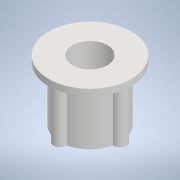
# Autodesk Inventor part: Tapa
Saved by Autodesk Inventor 2022 (Build 260153000, 153)
## iProperties
Created: 2022-08-23
Part Number: Tapa
Material: Generic
Document SubType Name: Modeling
Designer: David
Density: 1 g/cm^3
Appearance: Default
Author: David
Autodesk Inventor part; units mm, degrees
ref_plane "YZ Plane" through (0, 0, 0) normal (1, 0, 0) x (0, 1, 0)
ref_plane "XZ Plane" through (0, 0, 0) normal (0, 1, 0) x (-1, 0, 0)
ref_plane "XY Plane" through (0, 0, 0) normal (0, 0, 1) x (1, 0, 0)
sketch "Sketch8" plane through (0, 0, 0) normal (0, 1, 0) x (-1, 0, 0)
  circle A0 centre (0, 0) radius 13
  dimension "d25" = 26
  constraints: 1 centre point, 1 coincident
  measures "d25" diameter of A0
extrude "Extrusion8" add sketch "Sketch8" along normal blind 2
sketch "Sketch9" plane through (0, 0, 0) normal (0, -1, 0) x (1, 0, 0)
  circle A0 centre (0, 0) radius 9.5
  dimension "d28" = 19
  constraints: 1 centre point, 1 coincident
  measures "d28" diameter of A0
extrude "Extrusion9" add sketch "Sketch9" along normal blind 3
sketch "Sketch10" plane through (0, -3, 0) normal (0, -1, 0) x (1, 0, 0)
  circle A0 centre (0, 0) radius 9.5 projected
  circle A1 centre (-9.5, 0) radius 2
  line L0 (-18.2, 0) -> (18.2, 0) projected
  point P0 (-9.2895, -1.9889)
  point P1 (-9.2895, 1.9889)
  dimension "d31" = 4
  constraints: 1 centre point, 1 point on line, 2 other
  measures "d31" diameter of A1
extrude "Extrusion10" add sketch "Sketch10" against normal up to surface (3 mm away) contours A0 L0 A1 | A1 L0 A0 picked at (-10.0838, 0.5297) picked at (-10.0838, -0.5297)
pattern_circular "Circular Pattern2" count 4 over 360 about axis through (0, 0, 0) along (0, -1, 0) of "Extrusion10"
sketch "Sketch11" plane through (0, -3, 0) normal (0, -1, 0) x (1, 0, 0)
  circle A0 centre (0, 0) radius 5.5
  dimension "d41" = 11
  constraints: 1 centre point, 1 coincident
  measures "d41" diameter of A0
extrude "Extrusion11" cut sketch "Sketch11" against normal up to surface (5 mm away)
body "Solid2"
